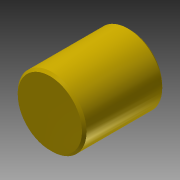
# Autodesk Inventor part: StandYellow
Saved by Autodesk Inventor 2014 SP1 (Build 180222100, 222)
## iProperties
Created: 2015-04-12
Part Number: StandYellow
Material: Wood (Oak)
Document SubType Name: Modeling
Designer: david
Density: 0.76 g/cm^3
Appearance: Smooth - Yellow
Mass: 144.01 g
Surface Area: 192.771 cm^2
Volume: 189.486 cm^3
Author: david
Autodesk Inventor part; units mm, degrees
ref_plane "YZ Plane" through (0, 0, 0) normal (1, 0, 0) x (0, 1, 0)
ref_plane "XZ Plane" through (0, 0, 0) normal (0, 1, 0) x (-1, 0, 0)
ref_plane "XY Plane" through (0, 0, 0) normal (0, 0, 1) x (1, 0, 0)
sketch "Sketch1" plane through (0, 0, 0) normal (0, 1, 0) x (-1, 0, 0)
  circle A0 centre (0, 0) radius 30
  dimension "d4" = 60
  constraints: 1 centre point, 1 coincident
  measures "d4" diameter of A0
extrude "Extrusion1" add sketch "Sketch1" along normal blind 70
sketch "Sketch2" plane through (0, 70, 0) normal (0, 1, 0) x (1, 0, 0)
  circle A0 centre (0, 0) radius 30 projected
  circle A1 centre (0, 0) radius 17.5
  dimension "d5" = 35
  constraints: 1 centre point, 1 coincident
  measures "d5" diameter of A1
extrude "Extrusion2" cut sketch "Sketch2" against normal blind 8 contours A1
chamfer "Chamfer1" distance 2 angle 45 2 edges at (30, 70, 0) (30, 0, 0)
body "Solid1"
